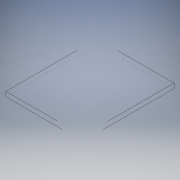
# Autodesk Inventor part: Extension Shelves
Saved by Autodesk Inventor 2016 (Build 200138000, 138)
## iProperties
Created: 2017-10-31
Part Number: Extension Shelves
Material: Wood (Oak)
Document SubType Name: Modeling
Designer: mathaetaes
Density: 0.76 g/cm^3
Appearance: White Oak - Natural Medium Gloss
Author: mathaetaes
Autodesk Inventor part; units mm, degrees
ref_plane "YZ Plane" through (0, 0, 0) normal (1, 0, 0) x (0, 1, 0)
ref_plane "XZ Plane" through (0, 0, 0) normal (0, 1, 0) x (-1, 0, 0)
ref_plane "XY Plane" through (0, 0, 0) normal (0, 0, 1) x (1, 0, 0)
sketch "Sketch1" plane through (0, 0, 0) normal (0, 1, 0) x (-1, 0, 0)
  line L0 (312.1225, 324.0216) -> (-94.2775, 324.0216)
  line L1 (-94.2775, 324.0216) -> (-94.2775, -158.5784)
  line L2 (-94.2775, -158.5784) -> (312.1225, -158.5784)
  line L3 (312.1225, -158.5784) -> (312.1225, 324.0216)
  point P0 (0, 0)
  dimension "d0" = 406.4
  dimension "d1" = 482.6
  constraints: 8 end point, 2 parallel, 1 horizontal, 1 perpendicular
  measures "d0" distance of L1.end L2.end
  measures "d1" distance of L0.end L1.end
extrude "Extrusion1" add sketch "Sketch1" along normal blind 25.4
body "Solid1"
